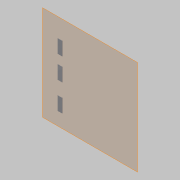
# Autodesk Inventor part: Navigation stripes
Saved by Autodesk Inventor 2015 (Build 190159000, 159)
## iProperties
Created: 2015-08-12
Part Number: Navigation stripes
Material: Generic
Document SubType Name: Modeling
Designer: v2jovano
Density: 1 g/cm^3
Appearance: Default
Author: v2jovano
Autodesk Inventor part; units mm, degrees
ref_plane "YZ Plane" through (0, 0, 0) normal (1, 0, 0) x (0, 1, 0)
ref_plane "XZ Plane" through (0, 0, 0) normal (0, 1, 0) x (-1, 0, 0)
ref_plane "XY Plane" through (0, 0, 0) normal (0, 0, 1) x (1, 0, 0)
ref_plane "Work Plane1" through (0, 0, 0) normal (0, 0, 1) x (1, 0, 0)
sketch "Sketch1" plane through (0, 0, 0) normal (0, 0, 1) x (1, 0, 0)
  line L0 (-914.4, -406.4) -> (-914.4, 406.4) projected
  line L1 (-914.4, 1219.2) -> (-914.4, 406.4) projected
  line L2 (-914.4, -1219.2) -> (-914.4, -406.4) projected
  line L3 (-914.4, 812.8) -> (-787.4, 812.8)
  line L4 (-787.4, 812.8) -> (-787.4, 431.8)
  line L5 (-787.4, 431.8) -> (-914.4, 431.8)
  line L6 (-914.4, 431.8) -> (-914.4, 812.8)
  line L7 (-914.4, 177.8) -> (-787.4, 177.8)
  line L8 (-787.4, 177.8) -> (-787.4, -203.2)
  line L9 (-787.4, -203.2) -> (-914.4, -203.2)
  line L10 (-914.4, -203.2) -> (-914.4, 177.8)
  line L11 (-914.4, -584.2) -> (-787.4, -584.2)
  line L12 (-787.4, -584.2) -> (-787.4, -965.2)
  line L13 (-787.4, -965.2) -> (-914.4, -965.2)
  line L14 (-914.4, -965.2) -> (-914.4, -584.2)
  line L15 (-1219.2, -1219.2) -> (1219.2, -1219.2) projected
  point P0 (0, 0)
  dimension "d0" = 127
  dimension "d1" = 254
  dimension "d2" = 381
  dimension "d3" = 381
  dimension "d4" = 381
  dimension "d5" = 254
  dimension "d6" = 381
  constraints: 24 end point, 6 parallel, 4 point on line, 3 horizontal, 3 perpendicular, 1 midpoint
  measures "d0" distance of L3.start L3.end
  measures "d1" distance between parallel lines of L15 L13
  measures "d2" distance of L11.end L12.end
  measures "d3" distance between parallel lines of L9 L11
  measures "d4" distance of L7.end L8.end
  measures "d5" distance between parallel lines of L7 L5
  measures "d6" distance of L3.end L4.end
extrude "Extrusion1" add sketch "Sketch1" along normal blind 6.35
body "Solid1"
